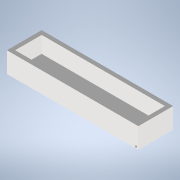
# Autodesk Inventor part: GiveBox
Saved by Autodesk Inventor 2021 (Build 250183000, 183)
## iProperties
Created: 2020-08-04
Part Number: GiveBox
Material: Generic
Document SubType Name: Modeling
Designer: karim
Density: 1 g/cm^3
Appearance: Default
Author: karim
Autodesk Inventor part; units mm, degrees
ref_plane "YZ Plane" through (0, 0, 0) normal (1, 0, 0) x (0, 1, 0)
ref_plane "XZ Plane" through (0, 0, 0) normal (0, 1, 0) x (-1, 0, 0)
ref_plane "XY Plane" through (0, 0, 0) normal (0, 0, 1) x (1, 0, 0)
sketch "Sketch1" plane through (0, 0, 0) normal (0, 1, 0) x (-1, 0, 0)
  line L0 (150, 32.4) -> (-150, 32.4)
  line L1 (-150, 32.4) -> (-150, -32.4)
  line L2 (-150, -32.4) -> (150, -32.4)
  line L3 (150, -32.4) -> (150, 32.4)
  line L4 (150, 32.4) -> (-150, -32.4) construction
  line L5 (-150, 32.4) -> (150, -32.4) construction
  line L6 (160, 42.4) -> (-160, 42.4)
  line L7 (-160, 42.4) -> (-160, -42.4)
  line L8 (-160, -42.4) -> (160, -42.4)
  line L9 (160, -42.4) -> (160, 42.4)
  point P0 (0, 0)
  dimension "d0" = 64.8
  dimension "d1" = 300
  dimension "d2" = 10
  dimension "d15" = 84.8
  constraints: 20 end point, 4 parallel, 2 midpoint, 2 perpendicular, 1 horizontal, 3 other
  measures "d0" distance of L0.end L1.end
  measures "d1" distance of L1.end L2.end
  measures "d2" distance between parallel lines of L3 L9
  measures "d15" distance of L8.end L6.start
extrude "Extrusion1" add sketch "Sketch1" along normal blind 10 contours L3 L2 L1 L0
extrude "Extrusion2" add sketch "Sketch1" along normal blind 50
sketch "Sketch2" plane through (160, 0, -42.4) normal (0, 0, -1) x (-1, 0, 0)
  point P0 (160, 0)
sketch "Sketch6" plane through (160, 0, -42.4) normal (0, 0, -1) x (-1, 0, 0)
  point P0 (160, 0)
sketch "Sketch7" plane through (160, 0, -42.4) normal (0, 0, -1) x (-1, 0, 0)
  point P0 (160, 0)
sketch "Sketch8" plane through (160, 0, -42.4) normal (0, 0, -1) x (-1, 0, 0)
  circle A0 centre (6.35, 4.7625) radius 3.175
  point P0 (160, 0)
  dimension "d12" = 6.35
  constraints: 1 centre point
  measures "d12" diameter of A0
extrude "Extrusion5" cut sketch "Sketch8" along normal mid plane 1000
body "Solid1"
